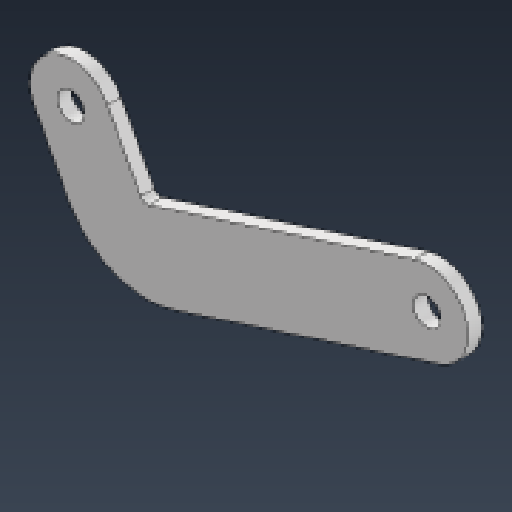
# Autodesk Inventor part: PLATE,LINK,REAR,INTAKE
Saved by Autodesk Inventor 2026 (Build 300175050, 175E)
## iProperties
Created: 2026-02-15
Part Number: PLATE,LINK,REAR,INTAKE
Material: Generic
Document SubType Name: Modeling
Designer: Jthib
Mass: 51.2814 g
Surface Area: 198.148 cm^2
Volume: 51.2814 cm^3
Density: 1 g/cm^3
Appearance: Default
Author: Jthib
Autodesk Inventor part; units mm, degrees
ref_plane "YZ Plane" through (0, 0, 0) normal (1, 0, 0) x (0, 1, 0)
ref_plane "XZ Plane" through (0, 0, 0) normal (0, 1, 0) x (-1, 0, 0)
ref_plane "XY Plane" through (0, 0, 0) normal (0, 0, 1) x (1, 0, 0)
sketch "Sketch1" plane through (0, 0, 0) normal (0, 0, 1) x (1, 0, 0)
  line L0 (-82.55, 0) -> (82.55, 0) construction
  arc A0 (-67.5221, 11.7074) -> (-97.5779, -11.7074) centre (-82.55, 0) ccw
  line L1 (-82.55, 0) -> (-58.8905, -30.3699) construction
  arc A1 (-58.8905, -30.3699) -> (-34.5194, -37.858) centre (-41.3579, -16.7112) ccw construction
  line L2 (-34.5194, -37.858) -> (82.55, 0) construction
  line L3 (76.6885, 18.1258) -> (-40.381, -19.7322)
  line L4 (-43.8625, -18.6625) -> (-68.2745, 12.6732)
  line L5 (-97.5779, -11.7074) -> (-73.9184, -42.0773)
  arc A2 (-73.9184, -42.0773) -> (-28.6579, -55.9838) centre (-41.3579, -16.7112) ccw
  line L6 (-28.6579, -55.9838) -> (88.4115, -18.1258)
  arc A3 (88.4115, -18.1258) -> (76.6885, 18.1258) centre (82.55, 0) ccw
  arc A4 (-43.8625, -18.6625) -> (-40.381, -19.7322) centre (-41.3579, -16.7112) ccw
  point P0 (0, 0)
  dimension "d1" = 38.1
  dimension "d2" = 165.1
  dimension "d14" = 22.225
  dimension "d15" = 110
  dimension "d16" = 50.8
  constraints: 16 end point, 10 point on circle, 7 tangent, 5 centre point, 1 concentric, 1 horizontal, 1 midpoint, 1 point on line, 3 other
  measures "d1" diameter of A0
  measures "d2" distance of L0.start L0.end
  measures "d14" radius of A1
  measures "d15" angle of L2 L1
  measures "d16" distance from line of L0.start L2
extrude "Extrusion1" add sketch "Sketch1" along normal mid plane 6.35
sketch "Sketch2" plane through (0, 0, 3.175) normal (0, 0, 1) x (1, 0, 0)
  arc A0 (-67.5221, 11.7074) -> (-97.5779, -11.7074) centre (-82.55, 0) ccw construction
  arc A1 (88.4115, -18.1258) -> (76.6885, 18.1258) centre (82.55, 0) ccw construction
  point P0 (0, 0)
  point P1 (-63.5, 19.05)
  point P2 (-63.5, -19.05)
  point P3 (63.5, -19.05)
  point P4 (63.5, 19.05)
  point P5 (-66.5399, 10.3236)
  point P6 (-97.8135, -11.3986)
  point P7 (73.7949, 16.9189)
  point P8 (82.55, -19.05)
  constraints: 2 coincident, 2 other
hole "Hole1" at (-82.55, 0, 3.175) at (82.55, 0, 3.175) direction (0, 0, -1) diameter 12.7 end through all start extended yes
body "Solid1"
